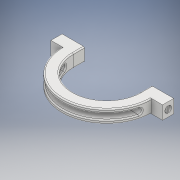
# Autodesk Inventor part: TopCircleArmHalf
Saved by Autodesk Inventor 2017 (Build 210142000, 142)
## iProperties
Created: 2017-02-18
Part Number: TopCircleArmHalf
Material: PBT Plastic
Document SubType Name: Modeling
Designer: aribu
Density: 1.31 g/cm^3
Appearance: Smooth - White
Author: aribu
Autodesk Inventor part; units mm, degrees
ref_plane "YZ Plane" through (0, 0, 0) normal (1, 0, 0) x (0, 1, 0)
ref_plane "XZ Plane" through (0, 0, 0) normal (0, 1, 0) x (-1, 0, 0)
ref_plane "XY Plane" through (0, 0, 0) normal (0, 0, 1) x (1, 0, 0)
sketch "Sketch1" plane through (0, 0, 0) normal (0, 0, 1) x (1, 0, 0)
  arc A0 (-30, 0) -> (30, 0) centre (0, 0) ccw
  arc A1 (-40, 0) -> (40, 0) centre (0, 0) ccw
  line L0 (-30, 0) -> (-30, 10)
  line L1 (30, 0) -> (30, 10)
  line L2 (-30, 10) -> (-50, 10)
  line L3 (-50, 10) -> (-50, 0)
  line L4 (-50, 0) -> (-40, 0)
  line L5 (30, 10) -> (50, 10)
  line L6 (50, 10) -> (50, 0)
  line L7 (50, 0) -> (40, 0)
  dimension "d0" = 60
  dimension "d1" = 80
  dimension "d12" = 20
  dimension "d13" = 20
  constraints: 16 end point, 4 perpendicular, 4 point on circle, 2 centre point, 2 coincident, 2 tangent, 1 horizontal, 1 vertical
  measures "d0" diameter of A0
  measures "d1" diameter of A1
  measures "d12" distance of L0.end L2.end
  measures "d13" distance of L1.end L5.end
extrude "Extrusion1" add sketch "Sketch1" along normal blind 12
sketch "Sketch2" plane through (50, 0, 0) normal (1, 0, 0) x (0, 0, -1)
  arc A0 (-3.5, -10) -> (-8.5, -10) centre (-6, -10) ccw
  line L0 (0, 10) -> (0, 0)
  line L1 (0, 0) -> (-10, 0)
  line L2 (-8.5, -10) -> (-8.5, -42.0097)
  line L3 (-8.5, -42.0097) -> (-3.5, -42.0097)
  line L4 (-3.5, -42.0097) -> (-3.5, -10)
  line L5 (0, 0) -> (-12, 0) projected
  line L6 (0, 10) -> (0, 0) projected
  dimension "d6" = 5
  dimension "d7" = 6
  dimension "d8" = 10
  dimension "d14" = 0
  dimension "d15" = 0
  dimension "d16" = 5
  constraints: 10 end point, 2 point on circle, 2 tangent, 1 centre point, 1 perpendicular, 1 vertical
  measures "d6" diameter of A0
  measures "d7" distance from line of L0 A0.centre
  measures "d8" distance from line of L1 A0.centre
  measures "d14" distance between parallel lines of L1 L5
  measures "d15" distance between parallel lines of L6 L0
  measures "d16" distance of L2.end L3.end
extrude "Extrusion2" cut sketch "Sketch2" against normal blind 90
fillet "Fillet1" radius 1 16 edges at (29.0474, -7.5, 6) (0, -30, 8.5) (-29.0474, -7.5, 6) (0, -30, 3.5) (-39.2906, -7.5, 5.9923) (0, -40, 8.5) (39.2906, -7.5, 5.9923) (0, -40, 3.5) (0, -40, 12) (0, -40, 0) (30, 5, 0) (-30, 5, 0) (0, -30, 0) (-30, 5, 12) (30, 5, 12) (0, -30, 12)
sketch "Sketch3" plane through (50, 0, 0) normal (1, 0, 0) x (0, 0, -1)
  line L0 (-12, 0) -> (-12, 10) projected
  line L1 (0, 10) -> (-12, 10) projected
  line L2 (-8.9139, 4.4) -> (-3.0861, 4.4)
  line L3 (-3.0861, 5.6) -> (-8.9139, 5.6)
  arc A0 (-8.9139, 4.4) -> (-3.0861, 4.4) centre (-6, 5) ccw
  arc A1 (-3.0861, 5.6) -> (-8.9139, 5.6) centre (-6, 5) ccw
  point P0 (0, 0)
  dimension "d18" = 6
  dimension "d19" = 5
  constraints: 4 end point, 4 point on circle, 2 centre point, 1 horizontal, 1 parallel
  measures "d18" distance from line of L0 A0.centre
  measures "d19" distance from line of A0.centre L1
extrude "Extrusion3" cut sketch "Sketch3" against normal blind 25
body "Solid1"
